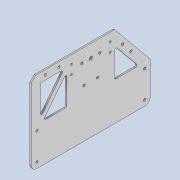
# Autodesk Inventor part: X Axis V Wheel Frame Machined
Saved by Autodesk Inventor 2022 (Build 260153000, 153)
## iProperties
Created: 2021-10-10
Part Number: X Axis V Wheel Frame Machined
Material: Generic
Document SubType Name: Modeling
Designer: Coy
Density: 1 g/cm^3
Appearance: Machined - Aluminum
Author: Coy
Autodesk Inventor part; units mm, degrees
ref_plane "YZ Plane" through (0, 0, 0) normal (1, 0, 0) x (0, 1, 0)
ref_plane "XZ Plane" through (0, 0, 0) normal (0, 1, 0) x (-1, 0, 0)
ref_plane "XY Plane" through (0, 0, 0) normal (0, 0, 1) x (1, 0, 0)
sketch "Sketch1" plane through (0, 0, 0) normal (1, 0, 0) x (0, 1, 0)
  line L0 (0, 0) -> (40, 0) construction
  line L1 (40, 0) -> (40, 66.5) construction
  line L2 (40, 66.5) -> (0, 66.5) construction
  line L3 (0, 66.5) -> (0, 0) construction
  line L4 (0, 66.5) -> (40, 66.5) construction
  line L5 (40, 66.5) -> (40, 86.5) construction
  line L6 (40, 86.5) -> (0, 86.5)
  line L7 (0, 86.5) -> (0, 66.5) construction
  line L8 (0, 0) -> (40, 0) construction
  line L9 (40, 0) -> (40, -20) construction
  line L10 (40, -20) -> (0, -20) construction
  line L11 (0, -20) -> (0, 0) construction
  line L12 (48.2, 61.45) -> (-8.2, 61.45) construction
  line L13 (-8.2, 61.45) -> (-8.2, 5.05) construction
  line L14 (-8.2, 5.05) -> (48.2, 5.05) construction
  line L15 (48.2, 5.05) -> (48.2, 61.45) construction
  line L16 (48.2, 33.25) -> (-8.2, 33.25) construction
  line L17 (40, 33.25) -> (0, 33.25) construction
  line L18 (43.57, 56.82) -> (-3.57, 56.82) construction
  line L19 (-3.57, 56.82) -> (-3.57, 9.68) construction
  line L20 (-3.57, 9.68) -> (43.57, 9.68) construction
  line L21 (43.57, 9.68) -> (43.57, 56.82) construction
  line L22 (43.57, 56.82) -> (48.2, 56.82) construction
  line L23 (43.57, 56.82) -> (43.57, 61.45) construction
  line L24 (-3.57, 9.68) -> (-8.2, 9.68) construction
  line L25 (-3.57, 9.68) -> (-3.57, 5.05) construction
  line L26 (40, -10) -> (0, -10) construction
  line L27 (40, 76.5) -> (0, 76.5) construction
  circle A0 centre (30, 76.5) radius 2.1
  circle A1 centre (10, 76.5) radius 2.1
  circle A2 centre (30, -10) radius 2.1
  circle A3 centre (10, -10) radius 2.1
  circle A4 centre (43.57, 56.82) radius 2.6 construction
  circle A5 centre (43.57, 9.68) radius 2.6 construction
  circle A6 centre (-3.57, 9.68) radius 2.6 construction
  circle A7 centre (-3.57, 56.82) radius 2.6 construction
  circle A8 centre (-25, 18.25) radius 11.08 construction
  circle A9 centre (-25, 18.25) radius 13 construction
  circle A10 centre (-25, 18.25) radius 2.5
  line L28 (-60, 153.25) -> (-60, -86.75) construction
  circle A11 centre (-60, -86.75) radius 2.6
  circle A12 centre (-60, 153.25) radius 2.6
  line L29 (-120.2, 153.25) -> (-120.2, -86.75) construction
  circle A13 centre (-120.2, -86.75) radius 2.6
  circle A14 centre (-120.2, 153.25) radius 2.6
  circle A15 centre (-60, -86.75) radius 12 construction
  circle A16 centre (-120.2, -86.75) radius 12 construction
  circle A17 centre (-120.2, 153.25) radius 12 construction
  circle A18 centre (-60, 153.25) radius 12 construction
  line L30 (-110, 482.7599) -> (-70, 482.7599) construction
  line L31 (-70, -517.2401) -> (-110, -517.2401) construction
  circle A19 centre (-25, 48.25) radius 2.5
  circle A20 centre (-25, 48.25) radius 11.08 construction
  circle A21 centre (-25, 48.25) radius 13 construction
  circle A22 centre (20, 33.25) radius 11.08 construction
  circle A23 centre (20, 33.25) radius 13 construction
  line L32 (-23.1873, 29.1807) -> (18.1873, 22.3193) construction
  line L33 (18.1873, 44.1807) -> (-23.1873, 37.3193) construction
  line L34 (-120.8333, -99.25) -> (-47.8333, -99.25)
  line L35 (-47.8333, 165.75) -> (-120.8333, 165.75)
  line L36 (-132.8333, 153.75) -> (-132.8333, -87.25)
  line L37 (-60, 153.25) -> (-120.2, 153.25) construction
  line L38 (-120.2, -86.75) -> (-60, -86.75) construction
  line L39 (-60, 153.25) -> (-60, 165.75) construction
  line L40 (-120.2, -86.75) -> (-120.2, -99.25) construction
  line L41 (48.3276, -20) -> (48.3276, 86.5)
  line L42 (17.6122, 86.5) -> (40, 86.5) construction
  arc A24 (-120.8333, 165.75) -> (-132.8333, 153.75) centre (-120.8333, 153.75) ccw
  arc A25 (-132.8333, -87.25) -> (-120.8333, -99.25) centre (-120.8333, -87.25) ccw
  line L43 (48.3276, -20) -> (-47.8333, -99.25)
  line L44 (-47.8333, 165.75) -> (-47.8333, -99.25) construction
  line L45 (-120.2, -86.75) -> (-132.8333, -86.75) construction
  line L46 (-60, 153.25) -> (-47.8333, 153.25) construction
  line L47 (-36.08, 48.25) -> (-36.08, 286.613) construction
  line L48 (-47.8333, 145.75) -> (-47.8333, 86.5)
  line L49 (-47.8333, 86.5) -> (16.8804, 86.5)
  line L50 (-47.8333, -73.3332) -> (16.8804, -20)
  line L51 (-47.8333, -20) -> (16.8804, -20)
  line L52 (-47.8333, -73.3332) -> (-47.8333, -20)
  line L53 (48.3276, 86.5) -> (48.3276, 165.75)
  line L54 (48.3276, 165.75) -> (-47.8333, 165.75)
  line L55 (-47.8333, 145.75) -> (28.3276, 145.75)
  line L56 (28.3276, 145.75) -> (28.3276, 86.5)
  line L57 (-47.8333, 145.75) -> (28.3276, 86.5) construction
  line L58 (-39.6904, 145.75) -> (28.3276, 92.8349)
  line L59 (-47.8333, 139.4151) -> (20.1847, 86.5)
  circle A26 centre (20, 33.25) radius 3.5
  line L60 (20, 33.25) -> (20, 13.25) construction
  line L61 (20, 33.25) -> (20, 53.25) construction
  circle A27 centre (20, 13.25) radius 2.6
  circle A28 centre (20, 53.25) radius 2.6
  point P0 (-132.8333, -99.25)
  point P1 (-132.8333, 165.75)
  point P2 (-47.8333, 139.8332)
  point P3 (0, 86.5)
  point P4 (0, 86.5)
  dimension "d181" = 22.16
  dimension "d156" = 40
  dimension "d157" = 66.5
  dimension "d158" = 40
  dimension "d159" = 20
  dimension "d160" = 40
  dimension "d161" = 20
  dimension "d162" = 56.4
  dimension "d163" = 56.4
  dimension "d164" = 0
  dimension "d165" = 8.2
  dimension "d166" = 47.14
  dimension "d167" = 47.14
  dimension "d168" = 4.2
  dimension "d169" = 20
  dimension "d170" = 10
  dimension "d171" = 10
  dimension "d172" = 20
  dimension "d173" = 4.2
  dimension "d174" = 4.2
  dimension "d175" = 4.2
  dimension "d176" = 5.2
  dimension "d177" = 5.2
  dimension "d178" = 5.2
  dimension "d179" = 5.2
  dimension "d182" = 26
  dimension "d183" = 5
  dimension "d184" = 240
  dimension "d185" = 60
  dimension "d186" = 5.2
  dimension "d187" = 5.2
  dimension "d188" = 5.2
  dimension "d189" = 5.2
  dimension "d190" = 60.2
  dimension "d191" = 24
  dimension "d192" = 24
  dimension "d193" = 24
  dimension "d194" = 24
  dimension "d195" = 40
  dimension "d196" = 1000
  dimension "d198" = 5
  dimension "d199" = 22.16
  dimension "d200" = 26
  dimension "d202" = 22.16
  dimension "d203" = 26
  dimension "d205" = 15
  dimension "d206" = 265
  dimension "d207" = 85
  dimension "d208" = 106.5
  dimension "d209" = 12
  dimension "d210" = 72.8333
  dimension "d212" = 53.25
  dimension "d213" = 85
  dimension "d214" = 132.5
  dimension "d215" = 60.2
  dimension "d216" = 20
  dimension "d217" = 20
  dimension "d218" = 5
  dimension "d219" = 5
  dimension "d220" = 7
  dimension "d221" = 20
  dimension "d222" = 20
  dimension "d223" = 5.2
  dimension "d224" = 5.2
  constraints: 124 end point, 28 centre point, 27 point on line, 20 coincident, 18 parallel, 17 perpendicular, 9 horizontal, 8 midpoint, 8 point on circle, 8 tangent, 6 vertical, 3 symmetric about line, 1 equal radius, 4 other
  measures "d156" distance of L2.end L1.end
  measures "d157" distance of L1.end L0.end
  measures "d158" distance of L5.end L6.end
  measures "d159" distance of L5.end L4.end
  measures "d160" distance of L9.end L10.end
  measures "d161" distance of L9.end L8.end
  measures "d162" distance of L14.end L13.end
  measures "d163" distance of L13.end L12.end
  measures "d164" distance between parallel lines of L17 L16
  measures "d165" distance between parallel lines of L15 L1
  measures "d166" distance of L20.end L18.start
  measures "d167" distance of L19.end L20.end
  measures "d168" diameter of A0
  measures "d169" distance of A1.centre A0.centre
  measures "d170" distance from line of L5 A0.centre
  measures "d171" distance from line of L9 A2.centre
  measures "d172" distance of A2.centre A3.centre
  measures "d173" diameter of A1
  measures "d174" diameter of A2
  measures "d175" diameter of A3
  measures "d176" diameter of A4
  measures "d177" diameter of A5
  measures "d178" diameter of A6
  measures "d179" diameter of A7
  measures "d182" diameter of A9
  measures "d183" diameter of A10
  measures "d184" distance of L28.start L28.end
  measures "d185" distance between parallel lines of L7 L28
  measures "d186" diameter of A11
  measures "d187" diameter of A12
  measures "d188" diameter of A13
  measures "d189" diameter of A14
  measures "d190" distance between parallel lines of L28 L29
  measures "d191" diameter of A15
  measures "d192" diameter of A16
  measures "d193" diameter of A17
  measures "d194" diameter of A18
  measures "d195" distance of L31.start L31.end
  measures "d196" distance of L30.end L31.start
  measures "d198" diameter of A19
  measures "d199" diameter of A20
  measures "d200" diameter of A21
  measures "d202" diameter of A22
  measures "d203" diameter of A23
  measures "d205" vertical distance of A22.centre A20.centre
  measures "d206" distance of point (-132.833, 165.75) point (-132.833, -99.25)
  measures "d207" distance of L35.start point (-132.833, 165.75)
  measures "d208" distance of L41.end L41.start
  measures "d209" radius of A24
  measures "d210" distance between parallel lines of L28 L36
  measures "d212" vertical distance of L41.end A22.centre
  measures "d213" distance of L34.end point (-132.833, -99.25)
  measures "d214" vertical distance of L35.start A23.centre
  measures "d215" distance of L37.start L37.end
  measures "d216" distance between parallel lines of L53 L56
  measures "d217" distance between parallel lines of L54 L55
  measures "d218" distance between parallel lines of L57 L58
  measures "d219" distance between parallel lines of L57 L59
  measures "d220" diameter of A26
  measures "d221" distance of L60.start L60.end
  measures "d222" distance of L60.start L61.end
  measures "d223" diameter of A27
  measures "d224" diameter of A28
extrude "Extrusion1" add sketch "Sketch1" along normal blind 3.175 contours L6 L59 L48 L55 L58 L56 | A25 L36 A24 L35 L54 L53 L41 L43 L34
sketch "Sketch4" plane through (3.175, 0, 0) normal (1, 0, 0) x (0, 0, -1)
  line L0 (20, 16.8804) -> (73.3332, -47.8333) projected
  line L1 (39.0796, -6.2705) -> (54.5136, 6.4492) construction
  line L2 (99.25, -47.8333) -> (20, 48.3276) construction
  line L3 (46.7966, 0.0893) -> (37.2568, 11.6648) construction
  line L4 (46.7966, 0.0893) -> (56.3364, -11.4861) construction
  circle A0 centre (37.2568, 11.6648) radius 2.6
  circle A1 centre (56.3364, -11.4861) radius 2.6
  line L5 (-145.75, 28.3276) -> (-92.8349, 28.3276) projected
  line L6 (-119.2924, 28.3276) -> (-119.2924, 48.3276) construction
  line L7 (20, 48.3276) -> (-165.75, 48.3276) construction
  line L8 (-119.2924, 38.3276) -> (-104.2924, 38.3276) construction
  line L9 (-119.2924, 38.3276) -> (-134.2924, 38.3276) construction
  circle A2 centre (-134.2924, 38.3276) radius 2.6
  circle A3 centre (-104.2924, 38.3276) radius 2.6
  point P0 (0, 0)
  point P1 (0, 0)
  dimension "d228" = 30
  dimension "d229" = 15
  dimension "d230" = 15
  dimension "d231" = 5.2
  dimension "d232" = 5.2
  dimension "d233" = 15
  dimension "d234" = 15
  dimension "d235" = 5.2
  dimension "d236" = 5.2
  dimension "d237" = 52.9151
  dimension "d238" = 26.4576
  constraints: 12 end point, 5 perpendicular, 4 centre point, 4 coincident, 3 midpoint, 3 point on line, 1 vertical
  measures "d228" distance from line of L0.start L1
  measures "d229" distance of L3.start L3.end
  measures "d230" distance of L3.start L4.end
  measures "d231" diameter of A0
  measures "d232" diameter of A1
  measures "d233" distance of L8.start L8.end
  measures "d234" distance of L8.start L9.end
  measures "d235" diameter of A3
  measures "d236" diameter of A2
  measures "d237" distance of L5.start L5.end
  measures "d238" distance from line of L5.end L6
extrude "Extrusion4" cut sketch "Sketch4" against normal through all
fillet "Fillet2" radius 3.175 11 edges at (1.5875, 28.3276, 92.8349) (1.5875, 20.1847, 86.5) (1.5875, -39.6904, 145.75) (1.5875, -47.8333, 139.4151) (1.5875, 16.8804, -20) (1.5875, 48.3276, -20) (1.5875, -47.8333, -20) (1.5875, -47.8333, -73.3332) (1.5875, -47.8333, -99.25) (1.5875, -47.8333, 86.5) (1.5875, 28.3276, 145.75)
chamfer "Chamfer1" distance 10 angle 45 1 edges at (1.5875, 48.3276, 165.75)
body "Solid1"
